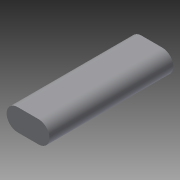
# Autodesk Inventor part: petite batterie
Saved by Autodesk Inventor 2013 (Build 170138000, 138)
## iProperties
Created: 2012-11-07
Part Number: petite batterie
Material: Générique
Document SubType Name: Modeling
Designer: Aegir
Density: 1 g/cm^3
Author: Aegir
Autodesk Inventor part; units mm, degrees
ref_plane "YZ Plane" through (0, 0, 0) normal (1, 0, 0) x (0, 1, 0)
ref_plane "XZ Plane" through (0, 0, 0) normal (0, 1, 0) x (-1, 0, 0)
ref_plane "XY Plane" through (0, 0, 0) normal (0, 0, 1) x (1, 0, 0)
sketch "Esquisse1" plane through (0, 0, 0) normal (0, 1, 0) x (-1, 0, 0)
  line L0 (0, 0) -> (-22, 0)
  line L1 (-22, 23) -> (0, 23)
  arc A0 (-22, 23) -> (-22, 0) centre (-22, 11.5) ccw
  arc A1 (0, 0) -> (0, 23) centre (0, 11.5) ccw
  dimension "d0" = 45
  dimension "d2" = 23
  constraints: 4 end point, 4 point on circle, 4 tangent, 2 centre point, 1 horizontal, 1 parallel
  measures "d2" distance between parallel lines of L0 L1
extrude "Extrusion1" add sketch "Esquisse1" along normal blind 130
